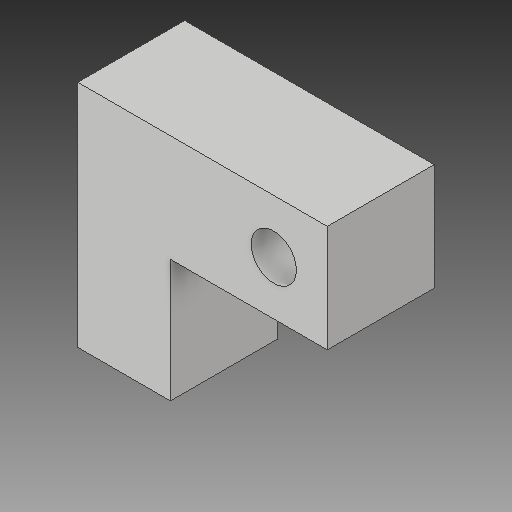
# Autodesk Inventor part: stand
Saved by Autodesk Inventor 2019 (Build 230136000, 136)
## iProperties
Created: 2019-11-28
Part Number: stand
Material: Generic
Document SubType Name: Modeling
Designer: felix
Density: 1 g/cm^3
Appearance: Default
Mass: 10754 g
Surface Area: 3749.1 cm^2
Volume: 10754 cm^3
Author: felix
Autodesk Inventor part; units mm, degrees
ref_plane "YZ Plane" through (0, 0, 0) normal (1, 0, 0) x (0, 1, 0)
ref_plane "XZ Plane" through (0, 0, 0) normal (0, 1, 0) x (-1, 0, 0)
ref_plane "XY Plane" through (0, 0, 0) normal (0, 0, 1) x (1, 0, 0)
sketch "Sketch1" plane through (0, 0, 0) normal (0, 0, 1) x (1, 0, 0)
  line L0 (-150, 322) -> (0, 322)
  line L1 (0, 322) -> (0, 0)
  line L2 (0, 0) -> (-150, 0)
  line L3 (-150, 0) -> (-150, 322)
  dimension "d0" = 150
  dimension "d1" = 322
  constraints: 8 end point, 2 parallel, 1 coincident, 1 horizontal, 1 perpendicular
  measures "d0" distance of L0.start L0.end
  measures "d1" distance of L2.end L0.start
extrude "Extrusion1" add sketch "Sketch1" along normal blind 150
sketch "Sketch2" plane through (0, 0, 150) normal (0, 0, 1) x (1, 0, 0)
  line L0 (0, 0) -> (0, 322) projected
  line L1 (0, 322) -> (-150, 322) projected
  point P0 (-75, 247)
  dimension "d4" = 75
  dimension "d5" = 75
  measures "d4" distance from line of L0 point (-75, 247)
  measures "d5" distance from line of L1 point (-75, 247)
hole "Hole1" at (-75, 247, 150) direction (0, 0, -1) diameter 63.5 end through all
sketch "Sketch3" plane through (-150, 0, 0) normal (-1, 0, 0) x (0, 0, 1)
  line L0 (0, 0) -> (0, 322) projected
  line L1 (150, 322) -> (150, 0) projected
  line L2 (0, 322) -> (150, 322)
  line L3 (150, 322) -> (150, 172)
  line L4 (150, 172) -> (0, 172)
  line L5 (0, 172) -> (0, 322)
  dimension "d13" = 150
  constraints: 8 end point, 2 parallel, 1 horizontal, 1 perpendicular, 1 point on line
  measures "d13" distance of L2.end L3.end
extrude "Extrusion2" add sketch "Sketch3" along normal blind 200
sketch "Sketch4" plane through (-150, 0, 0) normal (0, -1, 0) x (1, 0, 0)
  line L0 (150, 0) -> (0, 0) projected
  line L1 (0, 150) -> (150, 150) projected
  line L2 (0, 0) -> (150, 0)
  line L3 (150, 0) -> (150, 150)
  line L4 (150, 150) -> (0, 150)
  line L5 (0, 150) -> (0, 0)
  constraints: 8 end point, 2 parallel, 1 horizontal, 1 perpendicular
extrude "Extrusion3" cut sketch "Sketch4" against normal blind 172
sketch "Sketch5" plane through (-350, 172, 150) normal (0, -1, 0) x (1, 0, 0)
  line L0 (0, -150) -> (0, 0) projected
  line L1 (0, -150) -> (350, -150) projected
  line L2 (0, 0) -> (130, 0)
  line L3 (130, 0) -> (130, -150)
  line L4 (130, -150) -> (0, -150)
  line L5 (0, -150) -> (0, 0)
  dimension "d18" = 130
  constraints: 8 end point, 2 parallel, 1 horizontal, 1 perpendicular, 1 point on line
  measures "d18" distance of L3.end L4.end
extrude "Extrusion4" add sketch "Sketch5" along normal blind 172
body "Solid1"
